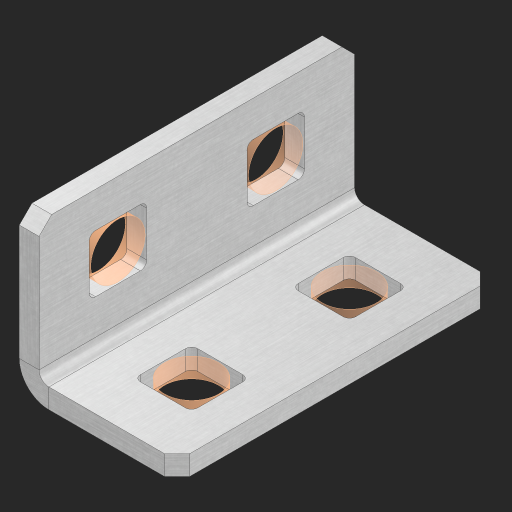
# Autodesk Inventor part: Alu C 1x2x1x35
Saved by Autodesk Inventor 2023 (Build 270158000, 158)
## iProperties
Created: 2022-07-28
Part Number: Alu C 1x2x1x35
Material: Generic
Document SubType Name: Sheet Metal
Designer: ylu12
Density: 1 g/cm^3
Sheet Metal Rule: Default
Appearance: Aluminum
Author: ylu12
Autodesk Inventor part; units mm, degrees
ref_plane "YZ Plane" through (0, 0, 0) normal (1, 0, 0) x (0, 1, 0)
ref_plane "XZ Plane" through (0, 0, 0) normal (0, 1, 0) x (-1, 0, 0)
sketch "Sketch1" plane through (0, 0, 0) normal (0, 1, 0) x (-1, 0, 0)
  line L0 (-6.35, 0) -> (6.35, 0)
  line L1 (6.35, 0) -> (6.35, -25.4)
  line L2 (6.35, -25.4) -> (-6.35, -25.4)
  line L3 (-6.35, -25.4) -> (-6.35, 0)
  line L4 (6.35, 0) -> (-6.35, -25.4) construction
  point P0 (0, 0)
  point P1 (0, 0)
  dimension "d0" = 12.7
  dimension "d1" = 25.4
  measures "d0" distance of L1.end L2.end
  measures "d1" distance of L0.end L1.end
extrude "Plate1" add sketch "Sketch1" along normal blind 1.5875
sketch "Sketch2" plane through (-4.7625, 0, 0) normal (-1, 0, 0) x (0, -1, 0)
  line L0 (0, -25.4) -> (0, 0)
  line L1 (0, 0) -> (-12.7, 0)
  line L2 (-12.7, 0) -> (-12.7, -25.4)
  line L3 (-12.7, -25.4) -> (0, -25.4)
  constraints: 6 end point, 1 horizontal, 1 perpendicular, 1 vertical
edge flange "Flanges" height 12.7 angle 90 thickness 1.5875 bend radius 0.7937 thickness toward (-1, 0, 0) relief tear relief width 1.5875 relief depth 0.7937 edges at (-6.35, 1.5875, -12.7) wall of the first edge with corners at (-4.7625, 0, -25.4) (-4.7625, 0, 0) (-4.7625, 12.7, 0) (-4.7625, 12.7, -25.4)
bend "Bend1"
corner "Corner1"
sketch "Sketch8" plane through (0, 0, 0) normal (0, -1, 0) x (1, 0, 0)
  line L0 (6.35, 0) -> (-3.9687, 0) construction
  line L1 (2.9718, -4.0386) -> (-0.635, -4.0386)
  line L2 (-1.143, -4.5466) -> (-1.143, -8.1534)
  line L3 (-0.635, -8.6614) -> (2.9718, -8.6614)
  line L4 (3.4798, -8.1534) -> (3.4798, -4.5466)
  arc A0 (3.4798, -4.5466) -> (2.9718, -4.0386) centre (2.9718, -4.5466) ccw
  arc A1 (2.9718, -8.6614) -> (3.4798, -8.1534) centre (2.9718, -8.1534) ccw
  arc A2 (-1.143, -8.1534) -> (-0.635, -8.6614) centre (-0.635, -8.1534) ccw
  arc A3 (-0.635, -4.0386) -> (-1.143, -4.5466) centre (-0.635, -4.5466) ccw
  line L5 (2.9718, -4.5466) -> (-0.635, -8.1534) construction
  line L6 (6.35, -25.4) -> (6.35, 0) construction
  point P0 (0, 0)
  point P1 (-1.143, -8.6614)
  point P2 (3.4798, -8.6614)
  point P3 (12.7, 0)
  point P4 (1.1684, -6.35)
  dimension "d49" = 4.6228
  dimension "d50" = 0.508
  dimension "d52" = 6.35
  dimension "d123" = 5.1816
  constraints: 10 end point, 8 point on circle, 8 tangent, 4 centre point, 4 point on line, 3 equal radius, 2 parallel, 2 perpendicular, 1 horizontal, 1 midpoint, 1 other
  measures "d49" distance of point (3.48, -8.661) point (-1.143, -8.661)
  measures "d50" radius of A0
  measures "d52" distance from line of L0 point (1.168, -6.35)
extrude "Body Stamp" cut sketch "Sketch8" against normal blind 1.5875
sketch "Sketch9" plane through (0, 0, 0) normal (0, -1, 0) x (1, 0, 0)
  arc A0 (3.4798, -4.5466) -> (2.9718, -4.0386) centre (2.9718, -4.5466) ccw construction
  arc A1 (-1.143, -8.1534) -> (-0.635, -8.6614) centre (-0.635, -8.1534) ccw construction
  line L0 (2.9718, -4.5466) -> (-0.635, -8.1534) construction
  circle A2 centre (1.1684, -6.35) radius 2.1844
  point P0 (0, 0)
  dimension "d55" = 4.3688
  constraints: 2 end point, 1 centre point, 1 midpoint
  measures "d55" diameter of A2
surface extrude "Body Circle" sketch "Sketch9" against normal up to surface (1.5875 mm away) shown yes curves A2
sketch "Body Pattern Sketch" plane through (0, 0, 0) normal (0, -1, 0) x (1, 0, 0)
  line L0 (1.1684, -6.35) -> (1.1684, 0) construction
  circle A0 centre (1.1684, -6.35) radius 2.1844 construction
  point P0 (1.1684, -19.05)
  dimension "d133" = 12.7
  constraints: 2 end point, 2 vertical, 1 coincident, 1 other
  measures "d133" distance of L0.start point (1.168, -19.05)
pattern_sketch "Body Pattern" of "Body Stamp", "Body Circle" from (1.1684, 0, -6.35) copies at (1.1684, 0, -19.05)
sketch "Arc Length" plane through (19.05, 2.3812, 0) normal (0, 0, 1) x (1, 0, 0)
  line L0 (-25.4, 0) -> (-23.8125, 0) projected
  arc A0 (-25.4, 0) -> (-23.0187, -2.3813) centre (-23.0187, 0) ccw projected
  line L1 (-23.0187, -0.7938) -> (-23.0187, -2.3813) projected
  arc A1 (-23.8125, 0) -> (-23.0187, -0.7938) centre (-23.0187, 0) ccw projected
  point P0 (-19.05, -2.3812)
  dimension "d126" = 1.2468
  dimension "d127" = 3.7405
sketch "Sketch13" plane through (-6.35, 0, 419.1) normal (1, 0, 0) x (0, 0, -1)
  line L0 (480.568, 12.7) -> (482.6, 10.668)
  line L1 (482.6, 10.668) -> (484.632, 12.7)
  line L2 (480.568, 12.7) -> (484.632, 12.7)
  line L3 (482.6, 3.3973) -> (480.3372, 1.1344)
  line L4 (480.3372, 1.1344) -> (482.6, -1.1284)
  line L5 (482.6, -1.1284) -> (484.8628, 1.1344)
  line L6 (484.8628, 1.1344) -> (482.6, 3.3973)
  line L7 (482.6, 3.3973) -> (482.6, -1.1284) construction
  line L8 (482.6, 10.668) -> (482.6, 3.3973) construction
  line L9 (444.5, 12.7) -> (419.1, 12.7) projected
  line L10 (444.5, 2.3813) -> (419.1, 2.3813) construction
  line L11 (419.1, 12.7) -> (419.1, 2.3813) construction
  point P0 (444.5, -11.9062)
  point P1 (419.1, 0)
  dimension "d86" = 4.5256
  dimension "d128" = 2.032
  dimension "d129" = 1.016
  dimension "d130" = 63.5
  constraints: 19 end point, 6 perpendicular, 2 vertical, 1 collinear, 1 other
  measures "d86" distance of L3.start L4.end
  measures "d128" distance from line of L2 L0.end
  measures "d130" distance between parallel lines of L11 L8
feature "Notch" [suppressed]
pattern_linear "Notch Pattern" [suppressed]
ref_plane "Diagonal Plane" through (-4.7625, 1.5875, 0) normal (-0.7071068, 0.7071068, 0) x (0, 0, 1)
mirror "Everything Mirrored" about plane through (-4.7625, 1.5875, 0) normal (-0.7071068, 0.7071068, 0) of "Body Stamp", "Body Circle", "Body Pattern"
chamfer "End Chamfer" distance 1.016 angle 45 4 edges at (-5.5562, 12.7, -25.4) (-5.5562, 12.7, 0) (6.35, 0.7937, 0) (6.35, 0.7937, -25.4)
equation "\"d1\" = 12.7 * Length"
equation "\"d53\" = Thickness"
equation "\"d89\" = Thickness"
equation "\"d2\" = Thickness"
equation "\"d3\" = BendReliefWidth"
equation "\"d4\" = BendReliefDepth"
equation "\"d5\" = MinimumRemnant"
equation "\"d6\" = TransitionRadius"
equation "\"d10\" = CornerReliefSize"
equation "\"d11\" = GapSize"
equation "\"d12\" = JacobiRadiusSize"
equation "\"BendRadius\" = Thickness"
equation "\"BendReliefWidth\" = Thickness"
equation "\"BendReliefDepth\" = 0.5 * Thickness"
equation "\"CornerReliefSize\" = 4 * Thickness"
equation "\"MinimumRemnant\" = 2 * Thickness"
equation "\"TransitionRadius\" = BendRadius"
equation "\"JacobiRadiusSize\" = BendRadius"
equation "\"GapSize\" = Thickness"
equation "\"Length\" = 2"
equation "\"Thickness\" = 1.5875"
body "Solid1"
body "Srf91"
body "Srf92"
body "Srf856"
body "Srf1275"
body "Srf1276"
body "Srf1278"
